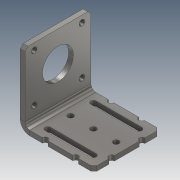
# Autodesk Inventor part: nema_support_techmakers
Saved by Autodesk Inventor 2017 (Build 210142000, 142)
## iProperties
Created: 2018-05-19
Part Number: nema_support_techmakers
Material: Steel, Alloy
Document SubType Name: Sheet Metal
Designer: Luiz Gustavo
Density: 7.73 g/cm^3
Sheet Metal Rule: Default_mm
Appearance: Semi-Polished
Author: Luiz Gustavo
Autodesk Inventor part; units mm, degrees
ref_plane "YZ Plane" through (0, 0, 0) normal (1, 0, 0) x (0, 1, 0)
ref_plane "XZ Plane" through (0, 0, 0) normal (0, 1, 0) x (-1, 0, 0)
ref_plane "XY Plane" through (0, 0, 0) normal (0, 0, 1) x (1, 0, 0)
sketch "Sketch1" plane through (0, 0, 0) normal (0, 0, 1) x (1, 0, 0)
  line L0 (-34, -32.5) -> (34, -32.5)
  line L1 (34, -32.5) -> (34, 32.5)
  line L2 (34, 32.5) -> (-34, 32.5)
  line L3 (-34, 32.5) -> (-34, -32.5)
  line L4 (-34, -32.5) -> (34, 32.5) construction
  line L5 (34, -32.5) -> (-34, 32.5) construction
  point P0 (0, 0)
  dimension "d0" = 68
  dimension "d1" = 65
  measures "d0" distance of L2.end L1.end
  measures "d1" distance of L1.end L0.end
extrude "Plate1" add sketch "Sketch1" along normal blind 4.76
sketch "Sketch2" plane through (-34, -32.5, 4.76) normal (-1, 0, 0) x (0, -1, 0)
  line L0 (-65, 0) -> (0, 0)
  line L1 (0, 0) -> (0, 68)
  line L2 (0, 68) -> (-65, 68)
  line L3 (-65, 68) -> (-65, 0)
  constraints: 6 end point, 1 horizontal, 1 perpendicular, 1 vertical
edge flange "Flange1" height 72.76 angle 90 thickness 4.76 bend radius 4.76 thickness toward (-1, 0, 0) relief tear relief width 4.76 relief depth 2.38 edges at (-34, 0, 4.76) wall of the first edge with corners at (-34, 32.5, 4.76) (-34, -32.5, 4.76) (-34, -32.5, 72.76) (-34, 32.5, 72.76)
bend "Bend1"
corner "Corner1"
sketch "Sketch3" plane through (0, 0, 4.76) normal (0, 0, 1) x (1, 0, 0)
  line L0 (-29.24, 32.5) -> (-29.24, -32.5) construction
  line L1 (34, -32.5) -> (-29.24, -32.5) construction
  line L2 (34, 32.5) -> (34, -32.5) construction
  line L3 (-29.24, 32.5) -> (34, 32.5) construction
  line L4 (-29.24, 32.5) -> (34, 32.5) projected
  circle A0 centre (-14, 32.5) radius 2.75
  circle A1 centre (16, 32.5) radius 2.75
  line L5 (34, 32.5) -> (34, -32.5) construction
  line L6 (34, 0) -> (-29.24, 0) construction
  line L7 (-29.24, 32.5) -> (-29.24, -32.5) construction
  arc A2 (-21.5, 25.25) -> (-21.5, 19.75) centre (-21.5, 22.5) ccw
  arc A3 (20.75, 22.5) -> (23.5, 19.75) centre (23.5, 22.5) ccw construction
  line L8 (-21.5, 22.5) -> (23.5, 22.5) construction
  line L9 (-21.5, 25.25) -> (23.5, 25.25)
  line L10 (23.5, 19.75) -> (-21.5, 19.75)
  arc A4 (-18.75, 22.5) -> (-21.5, 25.25) centre (-21.5, 22.5) ccw construction
  arc A5 (-21.5, 19.75) -> (-18.75, 22.5) centre (-21.5, 22.5) ccw construction
  arc A6 (23.5, 25.25) -> (20.75, 22.5) centre (23.5, 22.5) ccw construction
  arc A7 (23.5, 19.75) -> (23.5, 25.25) centre (23.5, 22.5) ccw
  circle A8 centre (34, 15) radius 2.75
  circle A9 centre (-14, -32.5) radius 2.75
  circle A10 centre (16, -32.5) radius 2.75
  arc A11 (-21.5, -19.75) -> (-21.5, -25.25) centre (-21.5, -22.5) ccw
  line L11 (-21.5, -25.25) -> (23.5, -25.25)
  line L12 (23.5, -19.75) -> (-21.5, -19.75)
  arc A12 (23.5, -25.25) -> (23.5, -19.75) centre (23.5, -22.5) ccw
  circle A13 centre (34, -15) radius 2.75
  line L13 (-21.5, 22.5) -> (-21.5, -22.5) construction
  line L14 (23.5, 22.5) -> (23.5, -22.5) construction
  line L15 (23.5, -22.5) -> (-21.5, -22.5) construction
  line L16 (1, -22.5) -> (1, 22.5) construction
  circle A14 centre (-21.5, 0) radius 2.75
  circle A15 centre (1, 0) radius 2.75
  circle A16 centre (23.5, 0) radius 2.75
  point P0 (0, 0)
  dimension "d13" = 5.5
  dimension "d14" = 30
  dimension "d15" = 18
  dimension "d16" = 5.5
  dimension "d17" = 45
  dimension "d18" = 10.5
  dimension "d19" = 45
  dimension "d20" = 30
  constraints: 20 end point, 17 centre point, 16 point on circle, 9 symmetric about line, 7 midpoint, 6 equal radius, 5 point on line, 4 tangent, 3 horizontal, 2 vertical, 1 perpendicular, 5 other
  measures "d13" diameter of A0
  measures "d14" distance of A1.centre A0.centre
  measures "d15" distance from line of L2 A1.centre
  measures "d16" diameter of A2
  measures "d17" distance of L8.end L8.start
  measures "d18" distance from line of L2 L8.end
  measures "d19" diameter of L8.end L6
  measures "d20" diameter of A8.centre L6
extrude "Cut1" cut sketch "Sketch3" against normal blind 4.76
sketch "Sketch4" plane through (-34, -32.5, 72.76) normal (1, 0, 0) x (0, 0, -1)
  line L0 (63.24, 0) -> (63.24, 65) construction
  line L1 (0, 65) -> (63.24, 65) construction
  line L2 (0, 65) -> (0, 0) construction
  line L3 (0, 0) -> (63.24, 0) construction
  line L4 (0, 65) -> (0, 0) construction
  line L5 (0, 32.5) -> (63.24, 32.5) construction
  circle A0 centre (30, 32.5) radius 15.25
  line L6 (53.55, 8.95) -> (6.45, 8.95) construction
  line L7 (6.45, 8.95) -> (6.45, 56.05) construction
  line L8 (6.45, 56.05) -> (53.55, 56.05) construction
  line L9 (53.55, 56.05) -> (53.55, 8.95) construction
  line L10 (53.55, 8.95) -> (6.45, 56.05) construction
  line L11 (6.45, 8.95) -> (53.55, 56.05) construction
  circle A1 centre (6.45, 8.95) radius 2.75
  circle A2 centre (6.45, 56.05) radius 2.75
  circle A3 centre (53.55, 56.05) radius 2.75
  circle A4 centre (53.55, 8.95) radius 2.75
  point P0 (72.76, 32.5)
  dimension "d23" = 30
  dimension "d24" = 30.5
  dimension "d25" = 47.1
  dimension "d26" = 5.5
  constraints: 14 end point, 5 centre point, 4 coincident, 4 midpoint, 3 equal radius, 2 parallel, 2 perpendicular, 1 horizontal, 1 point on line
  measures "d23" distance from line of A0.centre L2
  measures "d24" diameter of A0
  measures "d25" distance of L6.end L7.end
  measures "d26" diameter of A1
extrude "Cut2" cut sketch "Sketch4" against normal blind 4.76
chamfer "Corner Chamfer1" distance 3 angle 45 4 edges at (-36.38, 32.5, 72.76) (-36.38, -32.5, 72.76) (34, -32.5, 2.38) (34, 32.5, 2.38)
equation "\"d21\" = Thickness"
equation "\"d27\" = Thickness"
equation "\"d3\" = BendReliefWidth"
equation "\"d4\" = BendReliefDepth"
equation "\"d5\" = MinimumRemnant"
equation "\"d6\" = BendRadius"
equation "\"d9\" = BendRadius"
equation "\"d10\" = CornerReliefSize"
equation "\"d11\" = GapSize"
equation "\"d12\" = JacobiRadiusSize"
equation "\"BendRadius\" = Thickness"
equation "\"BendReliefWidth\" = Thickness"
equation "\"BendReliefDepth\" = 0.5 * Thickness"
equation "\"CornerReliefSize\" = 4 * Thickness"
equation "\"MinimumRemnant\" = 2 * Thickness"
equation "\"TransitionRadius\" = BendRadius"
equation "\"JacobiRadiusSize\" = BendRadius"
equation "\"GapSize\" = Thickness"
equation "\"d2\" = BendRadius"
equation "\"Thickness\" = 4.76"
body "Solid1"
